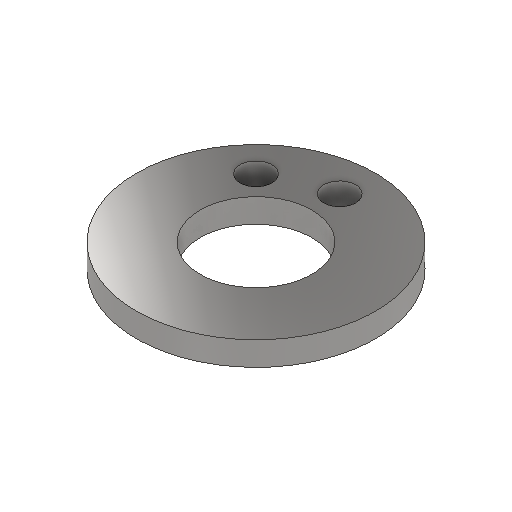
# Autodesk Inventor part: OringProbe_ring_pipe_adapter_4mm_version
Saved by Autodesk Inventor 2026.2 (Build 302298000, 298)
## iProperties
Created: 2022-11-25
Part Number: OringProbe_ring_pipe_adapter_4mm_version
Material: Stainless Steel, 440C
Document SubType Name: Modeling
Designer: kuzmin
Density: 7.75 g/cm^3
Appearance: 半つや出し
Author: kuzmin
Autodesk Inventor part; units mm, degrees
ref_plane "YZ Plane" through (0, 0, 0) normal (1, 0, 0) x (0, 1, 0)
ref_plane "XZ Plane" through (0, 0, 0) normal (0, 1, 0) x (-1, 0, 0)
ref_plane "XY Plane" through (0, 0, 0) normal (0, 0, 1) x (1, 0, 0)
sketch "Sketch1" plane through (0, 0, 0) normal (0, 1, 0) x (-1, 0, 0)
  circle A0 centre (0, 0) radius 15
  circle A1 centre (0, 0) radius 7
  dimension "d0" = 30
  dimension "d1" = 14
  dimension "d6" = 0
  constraints: 2 centre point, 2 coincident
  measures "d0" diameter of A0
  measures "d1" diameter of A1
  measures "d6" distance of A0.centre A1.centre
extrude "Extrusion1" add sketch "Sketch1" along normal blind 3
sketch "Sketch2" plane through (0, 3, 0) normal (0, 1, 0) x (1, 0, 0)
  circle A0 centre (0, 0) radius 15 projected
  line L0 (0, 0) -> (0, 10.5) construction
  circle A1 centre (0, 0) radius 10.5 construction
  line L1 (0, 0) -> (10.5, 0) construction
  dimension "d14" = 21
  dimension "d25" = 90
  constraints: 4 end point, 2 point on circle, 1 centre point, 1 coincident, 1 horizontal
  measures "d14" diameter of A1
  measures "d25" angle of L0 L1
hole "Hole1" at (0, 3, -10.5) direction (0, -1, 0) diameter 4 end through all
pattern_circular "Circular Pattern2" count 2 over 45 about axis through (0, 0, 0) along (0, 1, 0) of "Hole1"
body "Solid1"
